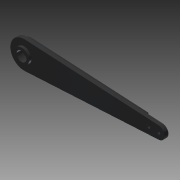
# Autodesk Inventor part: servo arm TGY-S8166M long
Saved by Autodesk Inventor 2013 (Build 170138000, 138)
## iProperties
Created: 2014-10-08
Part Number: servo arm TGY-S8166M long
Material: Generic
Document SubType Name: Modeling
Designer: Masta
Density: 1 g/cm^3
Author: Masta
Autodesk Inventor part; units mm, degrees
ref_plane "YZ Plane" through (0, 0, 0) normal (1, 0, 0) x (0, 1, 0)
ref_plane "XZ Plane" through (0, 0, 0) normal (0, 1, 0) x (-1, 0, 0)
ref_plane "XY Plane" through (0, 0, 0) normal (0, 0, 1) x (1, 0, 0)
sketch "Sketch1" plane through (0, 0, 0) normal (0, 1, 0) x (-1, 0, 0)
  arc A0 (-0.611111, -10.983012) -> (-0.611111, 10.983012) centre (0, 0) ccw
  line L0 (0, 0) -> (-108, 0) construction
  arc A1 (-108.277778, 4.992278) -> (-108.277778, -4.992278) centre (-108, 0) ccw
  line L1 (-0.611111, 10.983012) -> (-108.277778, 4.992278)
  line L2 (-0.611111, -10.983012) -> (-108.277778, -4.992278)
  circle A2 centre (0, 0) radius 6
  line L3 (-108.222222, 3.993822) -> (-0.555556, 9.984556)
  arc A3 (-0.555556, -9.984556) -> (-0.555556, 9.984556) centre (0, 0) ccw
  line L4 (-0.555556, -9.984556) -> (-108.222222, -3.993822)
  arc A4 (-108.222222, 3.993822) -> (-108.222222, -3.993822) centre (-108, 0) ccw
  line L5 (-95, -4.729527) -> (-95, 4.729527)
  point P0 (-100, 0)
  dimension "d0" = 22
  dimension "d1" = 108
  dimension "d2" = 10
  dimension "d3" = 8
  dimension "d6" = 12
  dimension "d7" = 1
  dimension "d8" = 13
  constraints: 12 end point, 8 point on circle, 5 centre point, 5 coincident, 3 point on line, 2 symmetric about line, 2 tangent, 1 horizontal, 1 perpendicular, 3 other
  measures "d0" diameter of A0
  measures "d1" distance of L0.start L0.end
  measures "d2" diameter of A1
  measures "d3" distance of point (-100, 0) L0.end
  measures "d6" diameter of A2
  measures "d7" distance between parallel lines of L1 L3
  measures "d8" distance from line of L5 point (-108, 0)
extrude "Extrusion1" add sketch "Sketch1" against normal blind 3 contours L2 A1 L1 A0 | A2 | L3 L5 L4 A4 | L3 A3 L4 L5
sketch "Sketch1 outline for Extrusion2" plane through (0, 0, 0) normal (0, 1, 0) x (-1, 0, 0)
  arc A0 (-0.555556, -9.984556) -> (-0.555556, 9.984556) centre (0, 0) ccw
  line L0 (-95, -4.729527) -> (-0.555556, -9.984556)
  line L1 (-95, 4.729527) -> (-95, -4.729527)
  line L2 (-0.555556, 9.984556) -> (-95, 4.729527)
extrude "Extrusion2" add sketch "Sketch1 outline for Extrusion2" along normal blind 3 draft -20
extrude "Extrusion3" add sketch "Sketch1" against normal blind 5 contours A2
hole "Hole1" at (108, 0, 0) at (100, 0, 0) direction (0, -1, 0) diameter 2.8 end through all
hole "Hole2" at (0, -5, 0) direction (0, 1, 0) diameter 3.5 end through all
hole "Hole3" at (0, -5, 0) direction (0, 1, 0) diameter 8 depth 5
body "Solid1"
